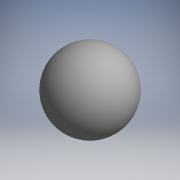
# Autodesk Inventor part: WA673SA Ball
Saved by Autodesk Inventor 2017.3 (Build 213256000, 256)
## iProperties
Part Number: WA673SA Ball
Material: Generic
Catalog Web Link: www.cadenas.de
Description: Six types ball-Metric system sizes
Vendor: NTN
Document SubType Name: Modeling
Designer: partserver
Manufacturer: NTN
Mass: 0.000366638 g
Surface Area: 0.0247728 cm^2
Volume: 0.000366638 cm^3
Density: 1 g/cm^3
Appearance: PSOLRGB-192-192-192
Category: PARTsolutions
Company: NTN
Title: WA673SA Ball
Author: Cadenas PARTsolutions
Comments: Metric system sizes
PSOL_IDENT_0: {$CADENAS_DATA\23d-libs\ntn\ball_roller_bearings\miniature_extra_small_bb\metric_system_sizes\mss_ba
PSOL_IDENT_1: ll.prj},175 {VTYP=3D},{NB=WA673SA Ball},{LINA=WA673SA Ball},{NN=Six types ball},{DATE=21.12.2021 04:
PSOL_IDENT_2: 23:04},{GEOMDATE=06.03.2020 10:07:36},{VERSION=},{LINEID=11430},{WBVAR=},{WBNUMERIC=}  {NB=WA673SA B
PSOL_IDENT_3: all},{LINA=WA673SA Ball},{KT=DUMMY},{IDNR=},{SD=3.0},{D=6},{B=2.0},{R=0.08},{ORDER=WA673SA},{CR=242}
PSOL_IDENT_4: ,{COR=94},{CRF=25},{CORF=9,5},{LSG=60 000},{LSO=71 000},{MASS=0.20},{ORDER1=673},{D1=7.2},{D2=7.2},{
PSOL_IDENT_5: C1=0.6},{C2=0.6},{WSS=WA673SA},{WDS=SSA},{UTWF=FL673},{FORSS=FLWA673SA},{FORDS=SSA},{DA1=3,6},{DA2=4
PSOL_IDENT_6: ,1},{DA=5,4},{RAS=0,08},{MASS1=0.26},{B1=2.5},{VERS=2},{X=1.5},{N=9},{O=14.13},{RB=0.444}
NB: WA673SA Ball
NN: Six types ball
NT: Metric system sizes
NBSYN: $ORDER. Ball
LINA: WA673SA Ball
CATALOG: NTN Corporation
SD: 3
D: 6
B: 2
R: 0.08
CR: 242
COR: 94
CRF: 25
CORF: 9,5
LSG: 60 000
LSO: 71 000
MASS: 0.2
ORDER1: 673
D1: 7.2
D2: 7.2
C1: 0.6
C2: 0.6
WSS: WA673SA
WDS: SSA
UTWF: FL673
FORSS: FLWA673SA
FORDS: SSA
DA1: 3,6
DA2: 4,1
DA: 5,4
RAS: 0,08
MASS1: 0.26
B1: 2.5
VERS: 2
SUPPLIER: NTN
ARTICLENO: WA673SA Ball
BOMINFO: WA673SA Ball
CREATOR: CADENAS GmbH
Autodesk Inventor part; units mm, degrees
sketch "Sketch_1" plane through (0, 0, 0) normal (0, 0, 1) x (1, 0, 0)
  line L0 (0.444, 0) -> (-0.444, 0)
  arc A0 (0.444, 0) -> (-0.444, 0) centre (0, 0) ccw
  line L1 (0.444, 0) -> (-0.444, 0)
  constraints: 4 end point, 2 point on circle, 1 centre point
revolve "Revolution1" add sketch "Sketch_1" angle 360 about axis through (0.444, 0, 0) along (1, 0, 0)
ref_plane "mss_ball_XY" through (0, 0, 0) normal (1, 0, 0) x (0, 0, -1)
ref_plane "mss_ball_YZ" through (0, 0, 0) normal (0, 0, -1) x (0, 1, 0)
ref_plane "mss_ball_ZX" through (0, 0, 0) normal (0, 1, 0) x (1, 0, 0)
body "Solid1"
